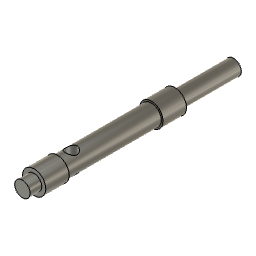
039424-01 MH Roller Driver Shaft (long) (Autodesk Fusion 360 design; units mm, degrees)
Autodesk Fusion 360 part; units mm, degrees
sketch "Profile" plane through (0, 0, 0) normal (0, 0, 1) x (1, 0, 0)
  line L0 (0, 0) -> (0, 85.725)
  line L1 (0, 0) -> (3.14325, 0)
  line L2 (3.14325, 0) -> (3.14325, 4.7244)
  line L3 (3.14325, 4.7244) -> (4.7498, 4.7244)
  line L4 (4.7498, 4.7244) -> (4.7498, 14.2494)
  line L5 (4.7498, 14.2494) -> (4.07035, 14.2494)
  line L6 (4.07035, 14.2494) -> (4.07035, 52.3494)
  line L7 (4.07035, 52.3494) -> (4.7498, 52.3494)
  line L8 (4.7498, 52.3494) -> (4.7498, 61.8744)
  line L9 (4.7498, 61.8744) -> (3.14325, 61.8744)
  line L10 (3.14325, 61.8744) -> (3.14325, 85.725)
  line L11 (3.14325, 85.725) -> (0, 85.725)
  dimension "d10" = 85.725
  dimension "d11" = 4.7244
  dimension "d12" = 9.525
  dimension "d14" = 3.14325
  dimension "d15" = 4.7498
  dimension "d16" = 4.07035
  dimension "d23" = 57.15
  constraint coincident L0.start L1.start
  constraint vertical L0
  constraint perpendicular L0 L1
  constraint perpendicular L1 L2
  constraint perpendicular L2 L3
  constraint perpendicular L3 L4
  constraint perpendicular L4 L5
  constraint perpendicular L5 L6
  constraint perpendicular L6 L7
  constraint perpendicular L7 L8
  constraint perpendicular L8 L9
  constraint perpendicular L9 L10
  constraint horizontal L11
  constraint collinear L4 L8
  constraint collinear L2 L10
  constraint equal L4 L8
  measures "d10" distance of L0.start L0.end
  measures "d12" distance of L3.end L4.end
  measures "d14" distance of L0 L2
  measures "d15" distance of L0 L4
  measures "d16" distance of L0 L6
  measures "d23" distance of L3 L9
revolve "Revolve1" add sketch "Profile" angle 360 about axis through (0, 0, 0) along (0, 1, 0)
sketch "ScrewHole" plane through (0, 85.725, 0) normal (0, 1, 0) x (-1, 0, 0)
  circle A0 centre (0, 0) radius 3.14325
  circle A1 centre (0, 0) radius 1.2192
  dimension "d21" = 2.4384
  constraint concentric A0 A1
  measures "d21" diameter of A1
extrude "Extrude1" cut sketch "ScrewHole" against normal blind 12.7 contours A1 picked at (0.177109, 0.267369)
sketch "TighteningHole" plane through (0, 0, 0) normal (0, 0, 1) x (1, 0, 0)
  line L0 (0, 0) -> (0, 19.80565) construction
  circle A0 centre (0, 19.80565) radius 2.38125
  line L1 (-4.7498, 14.2494) -> (4.7498, 14.2494)
  point P0 (-4.7498, 14.2494)
  point P1 (4.7498, 14.2494)
  dimension "d26" = 4.7625
  dimension "d29" = 5.55625
  constraint coincident L0.start origin
  constraint vertical L0
  measures "d26" diameter of A0
extrude "Extrude2" cut sketch "TighteningHole" along normal mid plane 8.1407
equation "OverallLength = 3 3/8\""
equation "BearingDiameter = 0.2475 in"
equation "RollerDiameter = 0.374 in"
equation "InsideDiameter = 0.3205 in"
equation "BearingLength = 0.1860 in"
equation "RollerLength = ( 3 / 8 ) * 1 in"
equation "d10 = OverallLength"
equation "d11 = BearingLength"
equation "d12 = RollerLength"
equation "d14 = BearingDiameter / 2"
equation "d15 = RollerDiameter / 2"
equation "d16 = InsideDiameter / 2"
equation "ScrewHoleDiameter = 0.0960 in" comment "Tap for #4-40 x 3/8 screw"
equation "ScrewHoleDepth = ( 1 / 2 ) * 1 in"
equation "d19 = -ScrewHoleDepth"
equation "d21 = ScrewHoleDiameter"
equation "RollerOutsideEdgeDistance = 2 1/4\""
equation "d23 = RollerOutsideEdgeDistance"
equation "TighteningHoleDistanceFromRoller = ( ( 1 / 32 ) * 1 in ) + ( TighteningHoleDiameter )"
equation "TighteningHoleDiameter = ( 3 / 16 ) * 1 in"
equation "d26 = TighteningHoleDiameter"
equation "d27 = InsideDiameter"
equation "d29 = TighteningHoleDistanceFromRoller"
